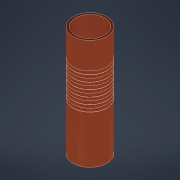
# Autodesk Inventor part: Test_Radiator
Saved by Autodesk Inventor 2022 (Build 260153000, 153)
## iProperties
Created: 2024-05-08
Part Number: Test_Radiator
Material: Generic
Document SubType Name: Modeling
Designer: jo_ki
Density: 1 g/cm^3
Appearance: Copper - Polished
Mass: 36.3453 g
Surface Area: 313.53 cm^2
Volume: 36.3453 cm^3
Author: jo_ki
Autodesk Inventor part; units mm, degrees
ref_plane "YZ Plane" through (0, 0, 0) normal (1, 0, 0) x (0, 1, 0)
ref_plane "XZ Plane" through (0, 0, 0) normal (0, 1, 0) x (-1, 0, 0)
ref_plane "XY Plane" through (0, 0, 0) normal (0, 0, 1) x (1, 0, 0)
sketch "Sketch6" plane through (0, 0, 0) normal (0, 1, 0) x (-1, 0, 0)
  circle A0 centre (0, 0) radius 16
  circle A1 centre (0, 0) radius 14
  dimension "d71" = 2
  dimension "d72" = 32
  constraints: 2 centre point, 2 coincident
  measures "d71" radial gap between concentric circles of A0 A1
  measures "d72" diameter of A0
extrude "Extrusion2" add sketch "Sketch6" along normal mid plane 103.75
sketch "Sketch7" plane through (0, 0, 0) normal (0, 0, 1) x (1, 0, 0)
  line L0 (-16, -51.875) -> (16, -51.875) projected
  line L1 (16, 51.875) -> (-16, 51.875) projected
  line L2 (16, 51.875) -> (-16, 51.875) projected
  line L3 (16, 51.875) -> (16, 26.875)
  line L4 (16, -51.875) -> (16, 51.875) projected
  line L5 (16, -51.875) -> (16, -6.875)
  line L6 (16, 26.875) -> (15.7, 26.875)
  line L7 (15.7, 26.875) -> (15.7, 23.625)
  line L8 (15.7, 23.625) -> (16, 23.625)
  line L9 (16, 20.775) -> (15.7, 20.775)
  line L10 (15.7, 20.775) -> (15.7, 17.525)
  line L11 (15.7, 17.525) -> (16, 17.525)
  line L12 (16, 17.525) -> (16, 20.775)
  line L13 (16, 14.675) -> (15.7, 14.675)
  line L14 (15.7, 14.675) -> (15.7, 11.425)
  line L15 (15.7, 11.425) -> (16, 11.425)
  line L16 (16, 11.425) -> (16, 14.675)
  line L17 (16, 8.575) -> (15.7, 8.575)
  line L18 (15.7, 8.575) -> (15.7, 5.325)
  line L19 (15.7, 5.325) -> (16, 5.325)
  line L20 (16, 5.325) -> (16, 8.575)
  line L21 (16, 2.475) -> (15.7, 2.475)
  line L22 (15.7, 2.475) -> (15.7, -0.775)
  line L23 (15.7, -0.775) -> (16, -0.775)
  line L24 (16, -0.775) -> (16, 2.475)
  line L25 (16, -3.625) -> (15.7, -3.625)
  line L26 (15.7, -3.625) -> (15.7, -6.875)
  line L27 (15.7, -6.875) -> (16, -6.875)
  line L28 (16, -6.875) -> (16, -3.625)
  line L29 (0, -72.625) -> (0, 72.625) projected
  point P0 (0, 0)
  dimension "d75" = 25
  dimension "d76" = 45
  dimension "d77" = 3.25
  dimension "d78" = 0.3
  dimension "d79" = 2.85
  dimension "d84" = 2.85
  dimension "d85" = 2.85
  dimension "d86" = 2.85
  dimension "d87" = 2.85
  constraints: 50 end point, 10 parallel, 7 horizontal, 6 collinear, 6 perpendicular, 5 point on line, 8 other
  measures "d75" distance of L1.start L3.end
  measures "d76" distance of L0.end L5.end
  measures "d77" distance of L6.end L7.end
  measures "d79" distance between parallel lines of L9 L8
  measures "d84" distance of L13.start L11.end
  measures "d85" distance of L17.start L15.end
  measures "d86" distance of L21.start L19.end
  measures "d87" distance of L25.start L23.end
revolve "Revolution2" cut sketch "Sketch7" angle 360 about axis through (0, -10, 0) along (0, 1, 0) contours L27 L26 L25 L4 | L4 L8 L7 L6 | L23 L22 L21 L4 | L4 L11 L10 L9 | L19 L18 L17 L4 | L4 L15 L14 L13
body "Solid2"
